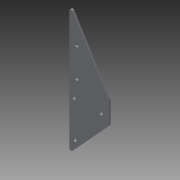
# Autodesk Inventor part: Ninja left cylinder support bracket
Saved by Autodesk Inventor 2013 (Build 170138000, 138)
## iProperties
Created: 2013-03-16
Part Number: Ninja left cylinder support bracket
Material: Generic
Document SubType Name: Modeling
Designer: Arpan
Density: 1 g/cm^3
Author: Arpan
Autodesk Inventor part; units mm, degrees
ref_plane "YZ Plane" through (0, 0, 0) normal (1, 0, 0) x (0, 1, 0)
ref_plane "XZ Plane" through (0, 0, 0) normal (0, 1, 0) x (-1, 0, 0)
ref_plane "XY Plane" through (0, 0, 0) normal (0, 0, 1) x (1, 0, 0)
sketch "Sketch1" plane through (0, 0, 0) normal (0, 0, 1) x (1, 0, 0)
  line L0 (69.85, 0) -> (69.85, 38.1)
  line L1 (69.85, 38.1) -> (0, 152.4)
  line L2 (0, 152.4) -> (0, 0)
  line L3 (69.85, 0) -> (0, -76.2)
  line L4 (0, -76.2) -> (0, 0)
  dimension "d1" = 38.1
  dimension "d2" = 152.4
  dimension "d24" = 76.2
  dimension "d25" = 69.85
  dimension "d26" = 69.85
  constraints: 10 end point, 1 collinear, 1 parallel, 1 vertical
  measures "d1" distance of L0.start L0.end
  measures "d2" distance of L1.end L2.end
  measures "d24" distance of L3.end L2.end
  measures "d25" distance between parallel lines of L2 L0
  measures "d26" distance of L2.end L0.start
extrude "Extrusion1" add sketch "Sketch1" along normal blind 3.175
sketch "Sketch2" plane through (0, 0, 3.175) normal (0, 0, 1) x (1, 0, 0)
  line L0 (0, 0) -> (69.85, 0) projected
  line L1 (69.85, 0) -> (69.85, 38.1) projected
  line L2 (0, 152.4) -> (0, -76.2) projected
  circle A0 centre (7.874, 12.7) radius 3.556
  circle A1 centre (55.626, 12.7) radius 3.556
  dimension "d5" = 7.112
  dimension "d6" = 7.112
  dimension "d7" = 12.7
  dimension "d8" = 12.7
  dimension "d9" = 14.224
  dimension "d11" = 7.874
  constraints: 2 centre point
  measures "d5" diameter of A0
  measures "d6" diameter of A1
  measures "d7" distance from line of L0 A0.centre
  measures "d8" distance from line of L0 A1.centre
  measures "d9" distance from line of L1 A1.centre
  measures "d11" distance from line of A0.centre L2
extrude "Extrusion2" cut sketch "Sketch2" against normal blind 25.4
fillet "Fillet1" radius 3.175 1 edges at (0, 152.4, 1.5875)
sketch "Sketch3" plane through (0, 0, 3.175) normal (0, 0, 1) x (1, 0, 0)
  line L0 (0, 141.1158) -> (0, -76.2) projected
  line L1 (0, 0) -> (69.85, 0) projected
  circle A0 centre (12.7, 94.9198) radius 3.3782
  circle A1 centre (12.7, 44.1198) radius 3.3782
  dimension "d15" = 6.7564
  dimension "d16" = 6.7564
  dimension "d17" = 12.7
  dimension "d18" = 12.7
  dimension "d19" = 44.1198
  dimension "d20" = 50.8
  constraints: 2 centre point
  measures "d15" diameter of A0
  measures "d16" diameter of A1
  measures "d17" distance from line of L0 A0.centre
  measures "d18" distance from line of L0 A1.centre
  measures "d19" distance from line of A1.centre L1
  measures "d20" distance of A0.centre A1.centre
extrude "Extrusion3" cut sketch "Sketch3" against normal blind 25.4
fillet "Fillet2" radius 3.175 2 edges at (69.85, 0, 1.5875) (69.85, 38.1, 1.5875)
fillet "Fillet3" radius 3.175 1 edges at (0, -76.2, 1.5875)
sketch "Sketch4" plane through (0, 0, 3.175) normal (0, 0, 1) x (1, 0, 0)
  line L0 (0, 141.1158) -> (0, -68.0377) projected
  circle A0 centre (12.7, 44.1198) radius 3.3782 projected
  circle A1 centre (9.525, -51.0773) radius 3.3782
  point P0 (0, 0)
  dimension "d28" = 6.7564
  dimension "d29" = 95.25
  dimension "d30" = 9.525
  constraints: 1 centre point
  measures "d28" diameter of A1
  measures "d29" distance of A0.centre A1.centre
  measures "d30" distance from line of L0 A1.centre
extrude "Extrusion4" cut sketch "Sketch4" against normal blind 25.4 contours A1
sketch "Sketch5" plane through (0, 0, 3.175) normal (0, 0, 1) x (1, 0, 0)
  circle A0 centre (12.7, 44.1198) radius 3.3782 projected
  circle A1 centre (12.7, 94.9198) radius 3.3782 projected
  point P0 (0, 0)
extrude "Extrusion5" cut sketch "Sketch5" against normal blind 25.4
body "Solid1"
